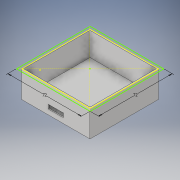
# Autodesk Inventor part: Cajapotenciometro_v1
Saved by Autodesk Inventor 2019 (Build 230136000, 136)
## iProperties
Created: 2020-06-11
Part Number: Cajapotenciometro_v1
Material: Genérico
Document SubType Name: Modeling
Designer: Samuel
Density: 1 g/cm^3
Appearance: Valor por defecto
Author: Samuel
Autodesk Inventor part; units mm, degrees
ref_plane "YZ Plane" through (0, 0, 0) normal (1, 0, 0) x (0, 1, 0)
ref_plane "XZ Plane" through (0, 0, 0) normal (0, 1, 0) x (-1, 0, 0)
ref_plane "XY Plane" through (0, 0, 0) normal (0, 0, 1) x (1, 0, 0)
sketch "Boceto1" plane through (0, 0, 0) normal (0, 1, 0) x (-1, 0, 0)
  line L0 (9, 7) -> (-56, 7)
  line L1 (-56, 7) -> (-56, -58)
  line L2 (-56, -58) -> (9, -58)
  line L3 (9, -58) -> (9, 7)
  point P0 (0, 0)
  dimension "d0" = 65
  dimension "d1" = 65
  constraints: 8 end point, 2 parallel, 1 horizontal, 1 perpendicular
  measures "d0" distance of L2.end L1.end
  measures "d1" distance of L1.end L0.end
extrude "Extrusión1" add sketch "Boceto1" along normal blind 3
sketch "Boceto2" plane through (0, 3, 0) normal (0, 1, 0) x (1, 0, 0)
  line L0 (-9, -7) -> (56, -7) projected
  line L1 (56, -7) -> (56, 58) projected
  line L2 (56, 58) -> (-9, 58) projected
  line L3 (-9, 58) -> (-9, -7) projected
  line L4 (-10, -8) -> (57, -8)
  line L5 (57, -8) -> (57, 59)
  line L6 (57, 59) -> (-10, 59)
  line L7 (-10, 59) -> (-10, -8)
  line L8 (-10, -8) -> (57, 59) construction
  line L9 (57, -8) -> (-10, 59) construction
  point P0 (0, 0)
  point P1 (23.5, 25.5)
  dimension "d4" = 67
  dimension "d5" = 67
  constraints: 12 end point, 2 midpoint, 2 parallel, 1 horizontal, 1 perpendicular
  measures "d4" distance of L6.end L5.end
  measures "d5" distance of L5.end L4.end
extrude "Extrusión2" add sketch "Boceto2" against normal blind 3
sketch "Boceto3" plane through (0, 3, 0) normal (0, 1, 0) x (1, 0, 0)
  line L0 (-10, -8) -> (57, -8) projected
  line L1 (57, -8) -> (57, 59) projected
  line L2 (57, 59) -> (-10, 59) projected
  line L3 (-10, 59) -> (-10, -8) projected
  line L4 (-9, -7) -> (56, -7)
  line L5 (56, -7) -> (56, 58)
  line L6 (56, 58) -> (-9, 58)
  line L7 (-9, 58) -> (-9, -7)
  line L8 (-9, -7) -> (56, 58) construction
  line L9 (56, -7) -> (-9, 58) construction
  point P0 (0, 0)
  point P1 (23.5, 25.5)
  dimension "d8" = 65
  dimension "d9" = 65
  constraints: 12 end point, 2 midpoint, 2 parallel, 1 horizontal, 1 perpendicular
  measures "d8" distance of L6.end L5.end
  measures "d9" distance of L5.end L4.end
extrude "Extrusión3" add sketch "Boceto3" along normal blind 23
sketch "Boceto4" plane through (-10, 0, 8) normal (0, 0, 1) x (1, 0, 0)
  line L0 (0, 26) -> (0, 0) projected
  line L1 (67, 0) -> (0, 0) projected
  line L2 (67, 0) -> (67, 26) projected
  line L3 (0, 26) -> (67, 26) projected
  line L4 (41, 9) -> (26, 9)
  line L5 (26, 9) -> (26, 5)
  line L6 (26, 5) -> (41, 5)
  line L7 (41, 5) -> (41, 9)
  line L8 (41, 9) -> (26, 5) construction
  line L9 (26, 9) -> (41, 5) construction
  point P0 (10, 0)
  point P1 (33.5, 7)
  constraints: 12 end point, 2 midpoint, 2 parallel, 1 horizontal, 1 perpendicular
extrude "Extrusión4" cut sketch "Boceto4" against normal blind 50 contours L7 L6 L5 L4
sketch "Boceto6" plane through (0, 26, 0) normal (0, 1, 0) x (1, 0, 0)
  line L0 (57, 59) -> (-10, 59) projected
  line L1 (57, -8) -> (57, 59) projected
  line L2 (-10, -8) -> (57, -8) projected
  line L3 (-10, 59) -> (-10, -8) projected
  line L4 (-12.5, 61.5) -> (59.5, 61.5)
  line L5 (59.5, 61.5) -> (59.5, -10.5)
  line L6 (59.5, -10.5) -> (-12.5, -10.5)
  line L7 (-12.5, -10.5) -> (-12.5, 61.5)
  line L8 (-12.5, 61.5) -> (59.5, -10.5) construction
  line L9 (59.5, 61.5) -> (-12.5, -10.5) construction
  point P0 (0, 0)
  point P1 (23.5, 25.5)
  dimension "d14" = 72
  dimension "d15" = 72
  constraints: 12 end point, 2 midpoint, 2 parallel, 1 horizontal, 1 perpendicular
  measures "d14" distance of L5.end L6.end
  measures "d15" distance of L4.end L5.end
